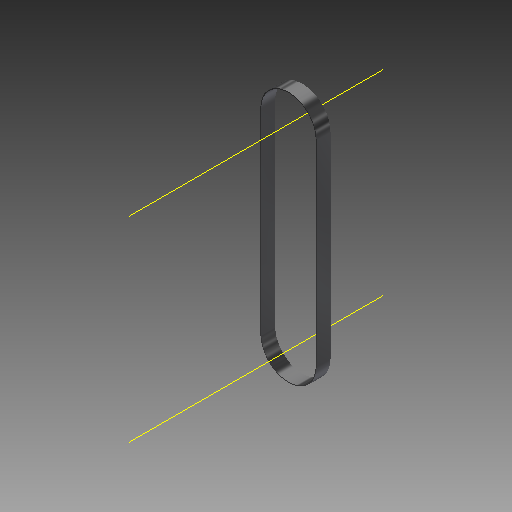
# Autodesk Inventor part: Synchronous Belt
Saved by Autodesk Inventor 2019.4 (Build 234330000, 330)
## iProperties
Created: 2019-12-14
Part Number: Synchronous Belt
Material: Rubber
Document SubType Name: Modeling
Designer: admin
Density: 1 g/cm^3
Appearance: Rubber - Black - Version 1.1
CustomPartVersion: 1
Author: admin
Autodesk Inventor part; units mm, degrees
sketch "Sketch Path" plane through (0, 0, 0) normal (0, 0, 1) x (1, 0, 0)
  arc A0 (46.831, 296.54) -> (-16.831, 296.54) centre (15, 296.54) ccw
  arc A1 (-16.831, 71.54) -> (46.831, 71.54) centre (15, 71.54) ccw
  line L0 (-16.831, 71.54) -> (-16.831, 296.54)
  line L1 (46.831, 296.54) -> (46.831, 71.54)
  constraints: 4 end point, 4 point on circle, 2 centre point
ref_plane "Cross Section Plane" through (-16.831, 296.54, 0) normal (0, -1, 0) x (0, 0, 1)
ref_plane "Work Plane2" through (15, 296.54, 0) normal (-1, 0, 0) x (0, 0, 1)
ref_plane "Work Plane3" through (15, 71.54, 0) normal (0.1564, 0.9877, 0) x (0, 0, 1)
sketch "Cross Section" plane through (-16.831, 296.54, 0) normal (0, -1, 0) x (0, 0, 1)
  line L0 (-8, 0.5) -> (8, 0.5)
  line L1 (8, 0.5) -> (8, -0.5)
  line L2 (8, -0.5) -> (-8, -0.5)
  line L3 (-8, -0.5) -> (-8, 0.5)
  line L4 (-8, 0) -> (8, 0) construction
  point P0 (0, 0)
  point P1 (0, 0)
  dimension "d0" = 16
  dimension "d4" = 0.5
  dimension "d5" = 0.5
  constraints: 10 end point, 3 midpoint, 2 parallel, 1 coincident, 1 horizontal, 1 perpendicular, 1 other
  measures "d0" distance between parallel lines of L1 L3
  measures "d4" distance between parallel lines of L2 L4
  measures "d5" distance between parallel lines of L4 L0
sweep "Belt" add profiles "Cross Section" path "Sketch Path"
equation "\"d0\" = da_B"
equation "\"d4\" = da_a"
equation "\"d5\" = da_a2"
equation "\"da_B\" = 16"
equation "\"da_pb\" = 5"
equation "\"da_a\" = 0.5"
equation "\"da_S\" = 2.65"
equation "\"da_Beta\" = 20deg"
equation "\"da_Ht\" = 1.2"
equation "\"da_H\" = 3.4"
equation "\"da_a2\" = 0.5"
body "Solid1"
